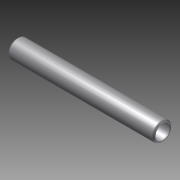
# Autodesk Inventor part: 007R-2.7390
Saved by Autodesk Inventor 2012 (Build 160160000, 160)
## iProperties
Created: 2013-01-17
Part Number: 007R-2.7390
Material: Default
Catalog Web Link: www.cadenas.de
Description: Tube-Original Line - Standard Air Cylinders
Vendor: BIMBA
Document SubType Name: Modeling
Designer: William
Manufacturer: BIMBA
Density: 1 g/cm^3
Category: PARTsolutions
Company: BIMBA
Title: 007R-2.7390
Author: Cadenas PARTsolutions
Comments: Original Line - Standard Air Cylinders
PSOL_IDENT_0: {\\10.0.0.242\data_v9\23d-libs\bimba\bimba\bimba_imperial\bimba_full_line\original_line_cylinders\st
PSOL_IDENT_1: andard_air_cylinders\tube.prj},190 {VTYP=3D},{NB=007R-2.7390},{LINA=007R-2.7390},{NN=Tube},{DATE=20.
PSOL_IDENT_2: 08.2011 07:16:50},{GEOMDATE=18.02.2011 00:00:00},{VERSION=},{LINEID=10},{LINESUBID=-1},{WBVAR=MNT,AC
PSOL_IDENT_3: TING,NR,L,FOURHOLES,SR}  {NB=007R-2.7390},{LINA=007R-2.7390},{KT=DUMMY},{PN=007R-2.7390},{BORE=0.312
PSOL_IDENT_4: 50000},{BOREPN=007},{MNT=},{MNTALG='' , 'Front Nose' , 'BF' , 'Front Block'},{ACTING=R},{ACTINGALG=
PSOL_IDENT_5: '' , 'Single Acting' , 'R' , 'Reverse/Double Acting' },{NR=},{NRALG= '' , 'N/A' },{L=2.7390},{OD=0.3
PSOL_IDENT_6: 590},{ODN=0.3590},{ODP=0.6050},{ODB=0.0000},{ID=0.3215},{DV=0.09400000},{LV=0.37500000},{LV1=0.03000
PSOL_IDENT_7: 000},{G=0.0220},{FOURHOLES=0},{AA=0.3250},{BB=0.0620},{SR=},{SRALG= 'C' , 'Carbon Steel Rod' , 'SR'
PSOL_IDENT_8: , '303 Stainless Steel Rod' , '' , '303 Stainless Steel Rod'}
CNS_NT: Original Line - Standard Air Cylinders
CNS_NB: 007R-2.7390
CNS_NBSYN: $PN.
CNS_LINA: 007R-2.7390
CNS_PN: 007R-2.7390
CNS_BORE: 5/16
CNS_BOREPN: 007
CNS_MNT: Front Nose
CNS_MNTALG: '' , 'Front Nose' , 'BF' , 'Front Block'
CNS_ACTING: Reverse/Double Acting
CNS_ACTINGALG: '' , 'Single Acting' , 'R' , 'Reverse/Double Acting'
CNS_NR: N/A
CNS_NRALG: '' , 'N/A'
CNS_L: 2.7390
CNS_OD: 0.3590
CNS_ODN: 0.3590
CNS_ODP: 0.6050
CNS_ODB: 0.0000
CNS_ID: 0.3215
CNS_DV: 0.09400000
CNS_LV: 0.37500000
CNS_LV1: 0.03000000
CNS_G: 0.0220
CNS_FOURHOLES: 0
CNS_AA: 0.3250
CNS_BB: 0.0620
CNS_SR: 303 Stainless Steel Rod
CNS_SRALG: 'C' , 'Carbon Steel Rod' , 'SR' , '303 Stainless Steel Rod' , '' , '303 Stainless Steel Rod'
SUPPLIER: BIMBA
ARTICLENO: 007R-2.7390
BOMINFO: 007R-2.7390
CREATOR: CADENAS GmbH
Autodesk Inventor part; units mm, degrees
sketch "Sketch_1" plane through (0, 0, 0) normal (0, 0, 1) x (1, 0, 0)
  line L0 (69.5706, 0) -> (0, 0)
  arc A0 (-0.445, 3.8695) -> (-0.445, 3.6899) centre (-0.3552, 3.7797) ccw
  line L1 (-0.445, 3.6899) -> (-0.2794, 3.5242)
  line L2 (-0.2794, 3.5242) -> (0, 3.5242)
  line L3 (0, 3.5242) -> (0.5588, 4.0831)
  line L4 (0.5588, 4.0831) -> (69.0118, 4.0831)
  line L5 (69.0118, 4.0831) -> (69.5706, 3.5242)
  line L6 (69.5706, 3.5242) -> (69.85, 3.5242)
  line L7 (69.85, 3.5242) -> (70.0156, 3.6899)
  arc A1 (70.0156, 3.6899) -> (70.0156, 3.8695) centre (69.9258, 3.7797) ccw
  line L8 (70.0156, 3.8695) -> (69.4895, 4.3956)
  arc A2 (69.4895, 4.3956) -> (69.0944, 4.5593) centre (69.0944, 4.0005) ccw
  line L9 (69.0944, 4.5593) -> (0.4763, 4.5593)
  arc A3 (0.4763, 4.5593) -> (0.0811, 4.3956) centre (0.4762, 4.0005) ccw
  line L10 (0.0811, 4.3956) -> (-0.445, 3.8695)
  constraints: 22 end point, 8 point on circle, 4 centre point
revolve "Revolution1" add sketch "Sketch_1" angle 360 about axis through (69.5706, 0, 0) along (1, 0, 0)
ref_plane "tube_front_XY" through (0, 0, 0) normal (1, 0, 0) x (0, 0, -1)
ref_plane "tube_front_YZ" through (0, 0, 0) normal (0, 0, -1) x (0, 1, 0)
ref_plane "tube_front_ZX" through (0, 0, 0) normal (0, 1, 0) x (1, 0, 0)
ref_plane "tube_rear_XY" through (69.5706, 0, 0) normal (1, 0, 0) x (0, 0, -1)
ref_plane "tube_rear_YZ" through (69.5706, 0, 0) normal (0, 0, -1) x (0, 1, 0)
ref_plane "tube_rear_ZX" through (69.5706, 0, 0) normal (0, 1, 0) x (1, 0, 0)
ref_plane "cp1_XY" through (34.7853, 4.5593, 0) normal (1, 0, 0) x (0, 0, -1)
ref_plane "cp1_YZ" through (34.7853, 4.5593, 0) normal (0, 0, -1) x (0, 1, 0)
ref_plane "cp1_ZX" through (34.7853, 4.5593, 0) normal (0, 1, 0) x (1, 0, 0)
ref_plane "cp2_XY" through (34.7853, 0, -4.5593) normal (1, 0, 0) x (0, 0, -1)
ref_plane "cp2_YZ" through (34.7853, 0, -4.5593) normal (0, 0, -1) x (0, 1, 0)
ref_plane "cp2_ZX" through (34.7853, 0, -4.5593) normal (0, 1, 0) x (1, 0, 0)
ref_plane "cp3_XY" through (34.7853, -4.5593, 0) normal (1, 0, 0) x (0, 0, -1)
ref_plane "cp3_YZ" through (34.7853, -4.5593, 0) normal (0, 0, -1) x (0, 1, 0)
ref_plane "cp3_ZX" through (34.7853, -4.5593, 0) normal (0, 1, 0) x (1, 0, 0)
ref_plane "cp4_XY" through (34.7853, 0, 4.5593) normal (1, 0, 0) x (0, 0, -1)
ref_plane "cp4_YZ" through (34.7853, 0, 4.5593) normal (0, 0, -1) x (0, 1, 0)
ref_plane "cp4_ZX" through (34.7853, 0, 4.5593) normal (0, 1, 0) x (1, 0, 0)
body "Solid1"
